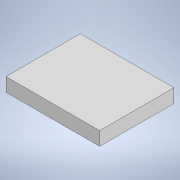
# Autodesk Inventor part: 77. Крышка верхняя
Saved by Autodesk Inventor 2021 (Build 250183000, 183)
## iProperties
Created: 2021-04-02
Part Number: 77. Крышка верхняя
Material: Типовые
Document SubType Name: Modeling
Designer: Данил
Density: 1 g/cm^3
Appearance: По умолчанию
Author: Данил
Autodesk Inventor part; units mm, degrees
ref_plane "YZ Plane" through (0, 0, 0) normal (1, 0, 0) x (0, 1, 0)
ref_plane "XZ Plane" through (0, 0, 0) normal (0, 1, 0) x (-1, 0, 0)
ref_plane "XY Plane" through (0, 0, 0) normal (0, 0, 1) x (1, 0, 0)
sketch "Эскиз5" plane through (0, 0, 0) normal (0, 1, 0) x (-1, 0, 0)
  line L0 (108, -126) -> (-139, -126)
  line L1 (-139, -126) -> (-139, 70)
  line L2 (-139, 70) -> (108, 70)
  line L3 (108, 70) -> (108, -126)
  point P0 (0, 0)
  point P1 (64, 58)
  point P2 (-104, 58)
  dimension "d19" = 64
  dimension "d20" = 58
  dimension "d21" = 203
  dimension "d22" = 12
  dimension "d23" = 184
  dimension "d24" = 168
  dimension "d25" = 212
  constraints: 8 end point, 2 parallel, 1 horizontal, 1 horizontal alignment, 1 perpendicular
  measures "d19" horizontal distance of point (64, 58) point (0, 0)
  measures "d20" vertical distance of point (64, 58) point (0, 0)
  measures "d21" distance from line of L1 point (64, 58)
  measures "d22" distance from line of L2 point (64, 58)
  measures "d23" distance from line of L0 point (64, 58)
  measures "d24" distance of point (-104, 58) point (64, 58)
  measures "d25" distance from line of L3 point (-104, 58)
extrude "Выдавливание2" add sketch "Эскиз5" along normal blind 36
